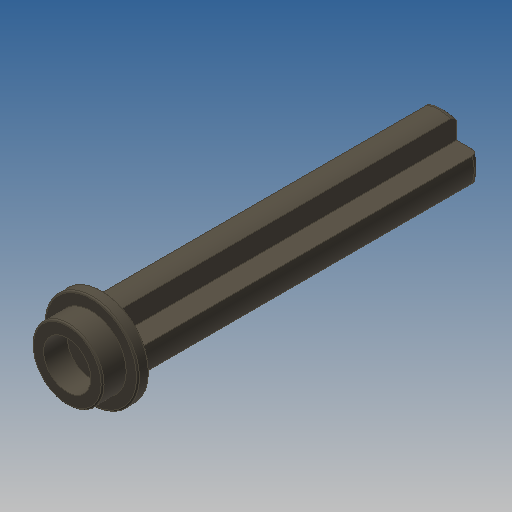
# Autodesk Inventor part: 6587-DkTan
Saved by Autodesk Inventor 2022.2 (Build 262287000, 287)
## iProperties
Created: 2014-06-05
Part Number: 6587-DkTan
Material: ABS Plastic
Document SubType Name: Modeling
Designer: D. Kohfeld
Density: 1.06 g/cm^3
Appearance: DarkTan
Mass: 0.349949 g
Surface Area: 5.35332 cm^2
Volume: 0.330141 cm^3
Author: D. Kohfeld
Autodesk Inventor part; units mm, degrees
ref_plane "YZ Plane" through (0, 0, 0) normal (1, 0, 0) x (0, 1, 0)
ref_plane "XZ Plane" through (0, 0, 0) normal (0, 1, 0) x (-1, 0, 0)
ref_plane "XY Plane" through (0, 0, 0) normal (0, 0, 1) x (1, 0, 0)
sketch "Sketch1" plane through (0, 0, 0) normal (0, 0, 1) x (1, 0, 0)
  circle A0 centre (0, 0) radius 2.4 construction
  line L0 (-0.8, 2.2627) -> (-0.8, 0.8)
  line L1 (-0.8, 0.8) -> (-2.2627, 0.8)
  line L2 (-2.2627, -0.8) -> (-0.8, -0.8)
  line L3 (-0.8, -0.8) -> (-0.8, -2.2627)
  line L4 (0.8, -2.2627) -> (0.8, -0.8)
  line L5 (0.8, -0.8) -> (2.2627, -0.8)
  line L6 (2.2627, 0.8) -> (0.8, 0.8)
  line L7 (0.8, 0.8) -> (0.8, 2.2627)
  arc A1 (0.8, 2.2627) -> (-0.8, 2.2627) centre (0, 0) ccw
  arc A2 (-2.2627, 0.8) -> (-2.2627, -0.8) centre (0, 0) ccw
  arc A3 (-0.8, -2.2627) -> (0.8, -2.2627) centre (0, 0) ccw
  arc A4 (2.2627, -0.8) -> (2.2627, 0.8) centre (0, 0) ccw
  dimension "d0" = 4.8
  dimension "d1" = 1.6
  constraints: 16 end point, 8 point on circle, 7 equal length, 4 centre point, 4 perpendicular, 3 parallel, 1 coincident, 1 vertical, 14 other
  measures "d1" distance between parallel lines of L0 L7
extrude "Extrusion1" add sketch "Sketch1" along normal mid plane 23.2
sketch "Sketch2" plane through (0, 0, 11.6) normal (0, 0, 1) x (1, 0, 0)
  arc A0 (0.8, 2.2627) -> (-0.8, 2.2627) centre (0, 0) ccw projected
  circle A1 centre (0, 0) radius 3.2
  dimension "d7" = 6.4
  constraints: 1 centre point, 1 coincident
  measures "d7" diameter of A1
extrude "Extrusion2" add sketch "Sketch2" along normal blind 0.8
sketch "Sketch3" plane through (0, 0, 12.4) normal (0, 0, 1) x (1, 0, 0)
  circle A0 centre (0, 0) radius 3.2 projected
  circle A1 centre (0, 0) radius 2.4
  circle A2 centre (0, 0) radius 1.6
  dimension "d10" = 4.8
  dimension "d11" = 3.2
  constraints: 2 centre point, 2 coincident
  measures "d10" diameter of A1
  measures "d11" diameter of A2
extrude "Extrusion3" add sketch "Sketch3" along normal blind 1.6 contours A1
sketch3d "Sketch4"
  constraints: 50 end point, 41 tangent, 38 point on circle, 19 centre point, 14 parallel, 13 equal radius, 10 horizontal, 4 collinear, 4 concentric, 3 point on line, 1 coincident, 1 midpoint, 1 other
feature "LEGO_SM:1" [suppressed]
fillet "Fillet1" radius 0.4 4 edges at (2.4, 0, -11.6) (0, 2.4, -11.6) (-2.4, 0, -11.6) (0, -2.4, -11.6)
fillet "Fillet1" radius 0.1 3 edges at (-2.4, 0, 14) (-3.2, 0, 12.4) (-3.2, 0, 11.6)
equation "\"d0\" = kd"
equation "\"d1\" = axlet"
equation "\"d2\" = 3 * lu - tsl"
equation "\"d7\" = tsd"
equation "\"d8\" = tsl"
equation "\"d10\" = kd"
equation "\"d11\" = rd"
equation "\"d12\" = knobh"
equation "\"d4\" = tf"
equation "\"d14\" = lf"
equation "\"lf\" = 0.1"
equation "\"tf\" = 0.4"
equation "\"kd\" = 4.8"
equation "\"axlet\" = 1.6"
equation "\"lu\" = 8"
equation "\"tsl\" = 0.8"
equation "\"tsd\" = 6.4"
equation "\"rd\" = 3.2"
equation "\"knobh\" = 1.6"
body "Solid1"
